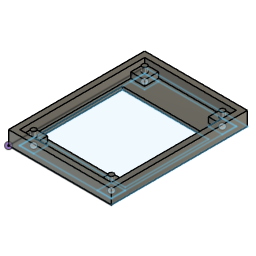
TFT Display Holder V2 v2 (Autodesk Fusion 360 design; units mm, degrees)
Autodesk Fusion 360 part; units mm, degrees
sketch "Sketch1" plane through (0, 0, 0) normal (0, 0, 1) x (1, 0, 0)
  line L0 (0, 0) -> (37, 0)
  line L1 (37, 0) -> (37, 49)
  line L2 (37, 49) -> (0, 49)
  line L3 (0, 49) -> (0, 0)
  line L4 (2, 2) -> (35, 2)
  line L5 (35, 2) -> (35, 47)
  line L6 (35, 47) -> (2, 47)
  line L7 (2, 47) -> (2, 2)
  circle A0 centre (4.5, 4.5) radius 0.8998
  circle A1 centre (32.5, 4.5) radius 0.9
  circle A2 centre (32.5, 44.5) radius 0.9002
  circle A3 centre (4.5, 44.5) radius 0.8999
  line L8 (3, 38) -> (34, 38)
  line L9 (34, 38) -> (34, 8)
  line L10 (34, 8) -> (3, 8)
  line L11 (3, 8) -> (3, 38)
  line L12 (2, 47) -> (7, 47)
  line L13 (7, 47) -> (7, 42)
  line L14 (7, 42) -> (2, 42)
  line L15 (2, 42) -> (2, 47)
  line L16 (35, 47) -> (30, 47)
  line L17 (30, 47) -> (30, 42)
  line L18 (30, 42) -> (35, 42)
  line L19 (35, 42) -> (35, 47)
  line L20 (35, 2) -> (30, 2)
  line L21 (30, 2) -> (30, 7)
  line L22 (30, 7) -> (35, 7)
  line L23 (35, 7) -> (35, 2)
  line L24 (2, 2) -> (7, 2)
  line L25 (7, 2) -> (7, 7)
  line L26 (7, 7) -> (2, 7)
  line L27 (2, 7) -> (2, 2)
  constraint horizontal L0
  constraint vertical L1
  constraint horizontal L2
  constraint vertical L3
  constraint coincident L0.start L3.end
  constraint horizontal L4
  constraint vertical L5
  constraint horizontal L6
  constraint vertical L7
  constraint horizontal L8
  constraint vertical L9
  constraint horizontal L10
  constraint vertical L11
  constraint horizontal L12
  constraint vertical L13
  constraint horizontal L14
  constraint vertical L15
  constraint horizontal L16
  constraint vertical L17
  constraint horizontal L18
  constraint vertical L19
  constraint horizontal L20
  constraint vertical L21
  constraint horizontal L22
  constraint vertical L23
  constraint horizontal L24
  constraint vertical L25
  constraint horizontal L26
  constraint vertical L27
extrude "Extrude1" add sketch "Sketch1" along normal blind 1 contours L0 L1 L2 L3 | L4 L7 L24 L25 L26 L27 | L4 L5 L6 L7 L13 L14 L17 L18 L21 L22 L25 L26 | L4 L5 L20 L21 L22 L23 | L6 L7 L12 L13 L14 L15 | L5 L6 L16 L17 L18 L19 | A0 | A1 | A2 | A3
extrude "Extrude2" cut sketch "Sketch1" along normal blind 4 contours L4 L7 L24 L25 L26 L27 | L4 L5 L20 L21 L22 L23 | L6 L7 L12 L13 L14 L15 | L5 L6 L16 L17 L18 L19 | A0 | A1 | A2 | A3
extrude "Extrude3" add sketch "Sketch1" along normal blind 4 contours L4 L7 L24 L25 L26 L27 | L4 L5 L20 L21 L22 L23 | L6 L7 L12 L13 L14 L15 | L5 L6 L16 L17 L18 L19 | A0 | A1 | A2 | A3
extrude "Extrude4" cut sketch "Sketch1" along normal blind 5 contours A0 | A1 | A2 | A3
extrude "Extrude5" add sketch "Sketch1" along normal blind 6 contours A0 | A1 | A2 | A3
extrude "Extrude6" cut sketch "Sketch1" along normal blind 4 contours L0 L1 L2 L3
extrude "Extrude7" add sketch "Sketch1" along normal blind 6 contours L0 L1 L2 L3
extrude "Extrude8" cut 4 faces at (4.5224, 2.5343, 4) (32.5224, 2.5342, 4) (4.5224, 42.5342, 4) (32.4776, 42.5341, 4) along direction (0, 0, -1) blind 1
extrude "Extrude9" cut 5 faces at (32.5668, 44.2075, 6) (0.6667, 17, 6) (4.65, 44.2402, 6) (4.7199, 4.7934, 6) (32.7134, 4.9094, 6) along direction (0, 0, -1) blind 1
